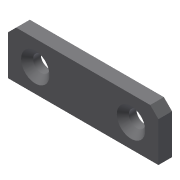
# Autodesk Inventor part: FixedJaw
Saved by Autodesk Inventor 2022 Beta2 (Build 260130000, 130) ContinuousBuild 0
## iProperties
Created: 2011-02-15
Part Number: FixedJaw
Material: Generic
Document SubType Name: Modeling
Designer: landrews
Density: 1 g/cm^3
Appearance: Light Gray
Author: landrews
Autodesk Inventor part; units mm, degrees
ref_plane "YZ Plane" through (0, 0, 0) normal (1, 0, 0) x (0, 1, 0)
ref_plane "XZ Plane" through (0, 0, 0) normal (0, 1, 0) x (-1, 0, 0)
ref_plane "XY Plane" through (0, 0, 0) normal (0, 0, 1) x (1, 0, 0)
sketch "Sketch1" plane through (0, 0, 0) normal (0, 1, 0) x (-1, 0, 0)
  line L0 (-38.5, 0) -> (38.5, 0) projected
  line L1 (27.5, 0) -> (-27.5, 0)
  line L2 (-27.5, 0) -> (-27.5, -17.5)
  line L3 (-27.5, -17.5) -> (27.5, -17.5)
  line L4 (27.5, -17.5) -> (27.5, 0)
  line L5 (0, -21) -> (0, 3.5) projected
  dimension "d8" = 17.5
  dimension "d22" = 55
  constraints: 8 end point, 2 parallel, 1 horizontal, 1 perpendicular, 1 point on line, 1 other
  measures "d8" distance between parallel lines of L3 L0
  measures "d22" distance of L2.end L3.end
extrude "Extrusion1" add sketch "Sketch1" along normal blind 5
sketch "Sketch2" plane through (0, 0, 0) normal (0, -1, 0) x (1, 0, 0)
  line L0 (-27.5, 0) -> (27.5, 0) projected
  line L1 (27.5, 0) -> (27.5, -17.5) projected
  line L2 (-27.5, -17.5) -> (-27.5, 0) projected
  point P0 (17.5, -9)
  point P1 (-17.5, -9)
  dimension "d9" = 9
  dimension "d23" = 10
  dimension "d24" = 10
  constraints: 1 horizontal alignment
  measures "d9" distance from line of L0 point (17.5, -9)
  measures "d23" distance from line of L2 point (-17.5, -9)
  measures "d24" distance from line of L1 point (17.5, -9)
hole "Hole1" at (17.5, 0, -9) at (-17.5, 0, -9) direction (0, 1, 0) diameter 6 end through all countersink diameter 10.4 countersink angle 90
chamfer "Chamfer1" distance 3 angle 45 2 edges at (-27.5, 2.5, 0) (27.5, 2.5, 0)
equation "\"d24\" = d23"
body "Solid1"
